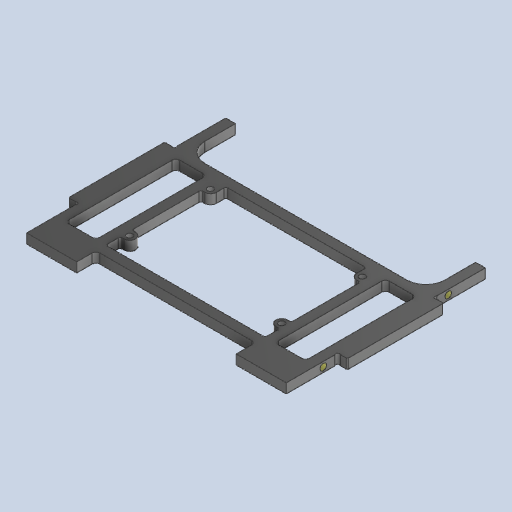
# Autodesk Inventor part: Cockpit_carrier_board_frame
Saved by Autodesk Inventor 2022 (Build 260153000, 153)
## iProperties
Part Number: Cockpit_carrier_board_frame
Material: アセタール樹脂、黒
Document SubType Name: Modeling
Designer: Masato Kubotera
Density: 1.425 g/cm^3
Appearance: 滑らか - 黒
Description: POM T5
Mass: 27.5617 g
Surface Area: 137.943 cm^2
Volume: 19.3415 cm^3
Author: Masato Kubotera
Autodesk Inventor part; units mm, degrees
ref_plane "YZ Plane" through (0, 0, 0) normal (1, 0, 0) x (0, 1, 0)
ref_plane "XZ Plane" through (0, 0, 0) normal (0, 1, 0) x (-1, 0, 0)
derived "Cockpit_side_frame.ipt"
sketch "スケッチ2" plane through (0, 0, 0) normal (0, 1, 0) x (-1, 0, 0)
  line L0 (-23.5, -22.5) -> (-28.5, -27.5)
  line L1 (-28.5, -27.5) -> (-28.5, -91)
  line L2 (-28.5, -91) -> (-23.5, -96)
  line L3 (-23.5, -96) -> (34.25, -96)
  line L4 (36.25, -98) -> (36.25, -131)
  line L5 (36.25, -131) -> (41.25, -136)
  line L6 (41.25, -136) -> (86.5, -136)
  line L7 (91.5, -131) -> (91.5, -20)
  line L8 (91.5, -20) -> (89, -17.5)
  line L9 (89, -17.5) -> (83.25, -17.5)
  line L10 (83.25, -17.5) -> (83.25, -21.0151)
  line L11 (81.7651, -22.5) -> (76.9849, -22.5)
  line L12 (75.5, -21.0151) -> (75.5, -17.5)
  line L13 (75.5, -17.5) -> (67.5, -17.5)
  line L14 (67.5, -17.5) -> (67.5, -21.0151)
  line L15 (66.0151, -22.5) -> (-23.5, -22.5)
  line L16 (-25.25, -25) -> (-20.25, -25) construction
  line L17 (-20.25, -25) -> (-20.25, -93.5) construction
  line L18 (-20.25, -93.5) -> (-25.25, -93.5) construction
  line L19 (-25.25, -93.5) -> (-25.25, -25) construction
  line L20 (-26, -25) -> (-25.25, -25) construction
  line L21 (-25.25, -93.5) -> (-26, -93.5) construction
  line L22 (-26, -93.5) -> (-26, -25) construction
  line L23 (-20.25, -93.5) -> (83.25, -93.5) construction
  line L24 (-20.25, -88.5) -> (83.25, -88.5) construction
  line L25 (83.25, -22.5) -> (83.25, -90.5) construction
  line L26 (83.25, -90.5) -> (88.25, -90.5) construction
  line L27 (88.25, -90.5) -> (88.25, -22.5) construction
  line L28 (83.25, -88.5) -> (83.25, -93.5) construction
  line L29 (83.25, -91) -> (88.25, -91) construction
  line L30 (88.25, -91) -> (88.25, -133.5) construction
  line L31 (83.25, -91) -> (83.25, -133.5) construction
  line L32 (83.25, -133.5) -> (88.25, -133.5) construction
  line L33 (38.75, -133.5) -> (38.75, -128.5) construction
  line L34 (38.75, -128.5) -> (38.75, -93.5) construction
  line L35 (43.75, -93.5) -> (43.75, -128.5) construction
  line L36 (38.75, -128.5) -> (43.75, -128.5) construction
  line L37 (41.25, -128.5) -> (41.25, -93.5) construction
  line L38 (38.75, -128.5) -> (82.1145, -128.5) construction
  line L39 (82.1145, -128.5) -> (82.1145, -133.5) construction
  line L40 (82.1145, -133.5) -> (38.75, -133.5) construction
  line L41 (38.75, -131) -> (82.1145, -131) construction
  line L42 (85.75, -91) -> (85.75, -133.5) construction
  circle A0 centre (85.75, -131) radius 2
  arc A1 (83.25, -128.5) -> (88.25, -128.5) centre (85.75, -131) ccw construction
  line L43 (83.25, -91) -> (-20.25, -91) construction
  line L44 (41.25, -111) -> (43.75, -111) construction
  line L45 (60.4322, -128.5) -> (60.4322, -131) construction
  line L46 (41.2, -115.5651) -> (41.2, -106.4349)
  line L47 (43.8, -107.05) -> (43.8, -114.95)
  line L48 (43.8, -117.05) -> (41.2, -104.95) construction
  line L49 (41.2, -117.05) -> (43.8, -104.95) construction
  line L50 (56.4822, -128.45) -> (64.3822, -128.45)
  line L51 (64.9973, -131.05) -> (55.8672, -131.05)
  line L52 (54.3822, -128.45) -> (66.4822, -131.05) construction
  line L53 (66.4822, -128.45) -> (54.3822, -131.05) construction
  line L54 (41.25, -105) -> (43.75, -105) construction
  line L55 (41.25, -117) -> (43.75, -117) construction
  arc A2 (42.6849, -104.95) -> (41.2, -106.4349) centre (41.9425, -105.6925) ccw
  arc A3 (43.8, -107.05) -> (43.8, -104.95) centre (43.8, -106) ccw
  arc A4 (41.2, -115.5651) -> (42.6849, -117.05) centre (41.9425, -116.3075) ccw
  arc A5 (43.8, -117.05) -> (43.8, -114.95) centre (43.8, -116) ccw
  line L56 (54.4322, -131) -> (54.4322, -128.5) construction
  line L57 (66.4322, -128.5) -> (66.4322, -131) construction
  arc A6 (54.3822, -129.5651) -> (55.8672, -131.05) centre (55.1247, -130.3075) ccw
  arc A7 (56.4822, -128.45) -> (54.3822, -128.45) centre (55.4322, -128.45) ccw
  arc A8 (64.9973, -131.05) -> (66.4822, -129.5651) centre (65.7398, -130.3075) ccw
  arc A9 (66.4822, -128.45) -> (64.3822, -128.45) centre (65.4322, -128.45) ccw
  line L58 (54.3822, -129.5651) -> (54.3822, -128.45)
  line L59 (66.4822, -128.45) -> (66.4822, -129.5651)
  line L60 (42.6849, -104.95) -> (43.8, -104.95)
  line L61 (43.8, -117.05) -> (42.6849, -117.05)
  circle A10 centre (48.4322, -131) radius 1.6
  line L62 (88.25, -22.5) -> (88.25, -17.5) construction
  line L63 (89, -17.5) -> (89, -90.5) construction
  line L64 (89, -90.5) -> (88.25, -90.5) construction
  line L65 (-13.5, -82.5) -> (-13.5, -61)
  arc A11 (-13.5, -82.5) -> (-11.5, -84.5) centre (-11.5, -82.5) ccw
  line L66 (45.5, -84.5) -> (-11.5, -84.5)
  arc A12 (45.5, -84.5) -> (47.5, -82.5) centre (45.5, -82.5) ccw
  line L67 (47.5, -61) -> (47.5, -82.5)
  arc A13 (47.5, -61) -> (45.5, -59) centre (45.5, -61) ccw
  line L68 (-11.5, -59) -> (45.5, -59)
  arc A14 (-11.5, -59) -> (-13.5, -61) centre (-11.5, -61) ccw
  line L69 (31.5, -88.5) -> (31.5, -91) construction
  line L70 (85.75, -22.5) -> (85.75, -90.5) construction
  circle A15 centre (85.75, -34) radius 1.6
  circle A16 centre (85.75, -34) radius 3
  circle A17 centre (85.75, -79) radius 3
  circle A18 centre (85.75, -79) radius 1.6
  line L71 (88.25, -22.5) -> (83.25, -22.5) construction
  arc A19 (88.25, -91) -> (83.25, -91) centre (85.75, -131) ccw construction
  circle A20 centre (48.4322, -131) radius 3
  circle A21 centre (41.25, -99) radius 1.6
  circle A22 centre (41.25, -99) radius 3
  line L72 (6.5, -88.5) -> (6.5, -91) construction
  line L73 (56.5, -88.5) -> (56.5, -91) construction
  line L74 (55.0651, -91.05) -> (7.9349, -91.05)
  line L75 (6.45, -89.5651) -> (6.45, -88.45)
  line L76 (8.55, -88.45) -> (54.45, -88.45)
  line L77 (56.55, -88.45) -> (56.55, -89.5651)
  line L78 (56.55, -91.05) -> (6.45, -88.45) construction
  line L79 (6.45, -91.05) -> (56.55, -88.45) construction
  arc A23 (8.55, -88.45) -> (6.45, -88.45) centre (7.5, -88.45) ccw
  arc A24 (6.45, -89.5651) -> (7.9349, -91.05) centre (7.1925, -90.3075) ccw
  arc A25 (55.0651, -91.05) -> (56.55, -89.5651) centre (55.8075, -90.3075) ccw
  arc A26 (56.55, -88.45) -> (54.45, -88.45) centre (55.5, -88.45) ccw
  line L80 (-20.25, -41) -> (83.25, -41) construction
  line L81 (83.25, -36) -> (-20.25, -36) construction
  line L82 (-20.25, -36) -> (-20.25, -41) construction
  line L83 (-20.25, -38.5) -> (83.25, -38.5) construction
  line L84 (31.5, -41) -> (31.5, -36) construction
  line L85 (55.0651, -35.95) -> (7.9349, -35.95)
  line L86 (7.9349, -41.05) -> (55.0651, -41.05)
  line L87 (56.55, -35.95) -> (6.45, -41.05) construction
  line L88 (6.45, -35.95) -> (55.5877, -40.952) construction
  arc A27 (7.9349, -35.95) -> (6.45, -37.4349) centre (7.1925, -36.6925) ccw
  arc A28 (6.45, -39.5651) -> (7.9349, -41.05) centre (7.1925, -40.3075) ccw
  arc A29 (56.55, -37.4349) -> (55.0651, -35.95) centre (55.8075, -36.6925) ccw
  arc A30 (55.0651, -41.05) -> (56.55, -39.5651) centre (55.8075, -40.3075) ccw
  line L89 (6.5, -41) -> (6.5, -36) construction
  line L90 (56.5, -36) -> (56.5, -41) construction
  line L91 (6.45, -37.4349) -> (6.45, -39.5651)
  line L92 (56.55, -39.5651) -> (56.55, -37.4349)
  circle A31 centre (-1, -38.5) radius 1.6
  circle A32 centre (-1, -38.5) radius 3
  circle A33 centre (64, -38.5) radius 1.6
  circle A34 centre (64, -38.5) radius 3
  line L93 (-25.25, -49.25) -> (-26, -49.25) construction
  line L94 (-25.25, -69.25) -> (-26, -69.25) construction
  line L95 (-26, -59.25) -> (-25.25, -59.25) construction
  line L96 (-22.75, -25) -> (-22.75, -93.5) construction
  arc A35 (66.0151, -22.5) -> (67.5, -21.0151) centre (66.7575, -21.7575) ccw
  arc A36 (75.5, -21.0151) -> (76.9849, -22.5) centre (76.2425, -21.7575) ccw
  line L97 (59.75, -22.5) -> (59.75, -32.5) construction
  line L98 (59.75, -32.5) -> (83.25, -32.5) construction
  line L99 (83.25, -32.5) -> (83.25, -22.5) construction
  line L100 (71.5, -17.5) -> (71.5, -32.5) construction
  line L101 (63.5, -22.5) -> (63.5, -17.5) construction
  line L102 (79.5, -22.5) -> (79.5, -17.5) construction
  circle A37 centre (-22.75, -31.75) radius 1.6
  circle A38 centre (-22.75, -31.75) radius 3
  circle A39 centre (-22.75, -86.75) radius 1.6
  circle A40 centre (-22.75, -86.75) radius 3
  line L103 (67.5, -22.5) -> (75.5, -22.5)
  line L104 (88.25, -17.5) -> (52.5, -17.5) construction
  line L105 (52.5, -17.5) -> (52.5, -22.5) construction
  circle A41 centre (85.75, -98.5) radius 1.475
  circle A42 centre (85.75, -103.5) radius 1.475
  circle A43 centre (85.75, -108.5) radius 1.475
  line L106 (48.25, -93.5) -> (78.75, -93.5)
  line L107 (80.75, -95.5) -> (80.75, -124)
  line L108 (78.75, -126) -> (48.25, -126)
  line L109 (46.25, -124) -> (46.25, -95.5)
  arc A44 (48.25, -93.5) -> (46.25, -95.5) centre (48.25, -95.5) ccw
  arc A45 (46.25, -124) -> (48.25, -126) centre (48.25, -124) ccw
  arc A46 (78.75, -126) -> (80.75, -124) centre (78.75, -124) ccw
  arc A47 (80.75, -95.5) -> (78.75, -93.5) centre (78.75, -95.5) ccw
  arc A48 (36.25, -98) -> (34.25, -96) centre (34.25, -98) ccw
  circle A49 centre (-13.5, -55) radius 1.75
  circle A50 centre (-13.5, -55) radius 2
  line L110 (77.85, -78.65) -> (68.65, -78.65) construction
  line L111 (68.65, -78.65) -> (68.65, -64.85) construction
  line L112 (68.65, -64.85) -> (77.85, -64.85) construction
  line L113 (77.85, -64.85) -> (77.85, -78.65) construction
  line L114 (77.85, -78.65) -> (68.65, -64.85) construction
  line L115 (68.65, -78.65) -> (77.85, -64.85) construction
  line L116 (67.95, -64.2) -> (78.55, -64.2) construction
  line L117 (78.55, -64.2) -> (78.55, -79.3) construction
  line L118 (78.55, -79.3) -> (67.95, -79.3) construction
  line L119 (67.95, -79.3) -> (67.95, -64.2) construction
  line L120 (67.95, -64.2) -> (78.55, -79.3) construction
  line L121 (78.55, -64.2) -> (67.95, -79.3) construction
  line L122 (69.3849, -64.15) -> (77.1151, -64.15)
  line L123 (78.6, -65.6349) -> (78.6, -77.8651)
  line L124 (78.6, -79.35) -> (67.9, -64.15) construction
  line L125 (67.9, -79.35) -> (78.6, -64.15) construction
  line L126 (77.9, -78.7) -> (68.6, -64.8) construction
  line L127 (68.6, -78.7) -> (77.9, -64.8) construction
  arc A51 (69.3849, -64.15) -> (67.9, -65.6349) centre (68.6425, -64.8925) ccw
  arc A52 (70.0849, -64.8) -> (68.6, -66.2849) centre (69.3425, -65.5425) ccw
  line L128 (67.9, -71.75) -> (78.6, -71.75) construction
  line L129 (73.25, -64.15) -> (73.25, -78.7063) construction
  arc A53 (78.6, -65.6349) -> (77.1151, -64.15) centre (77.8575, -64.8925) ccw
  arc A54 (77.9, -66.2849) -> (76.4151, -64.8) centre (77.1575, -65.5425) ccw
  arc A55 (68.6, -77.2151) -> (70.0849, -78.7) centre (69.3425, -77.9575) ccw
  arc A56 (67.9, -77.8651) -> (69.3849, -79.35) centre (68.6425, -78.6075) ccw
  arc A57 (76.4151, -78.7) -> (77.9, -77.2151) centre (77.1575, -77.9575) ccw
  arc A58 (77.1151, -79.35) -> (78.6, -77.8651) centre (77.8575, -78.6075) ccw
  line L130 (70.0849, -64.8) -> (76.4151, -64.8)
  line L131 (77.9, -66.2849) -> (77.9, -77.2151)
  line L132 (67.9, -77.8651) -> (67.9, -65.6349)
  line L133 (68.6, -77.2151) -> (68.6, -66.2849)
  line L134 (76.4151, -78.7) -> (70.0849, -78.7)
  line L135 (77.1151, -79.35) -> (69.3849, -79.35)
  line L136 (-13.5, -71.75) -> (47.5, -71.75) construction
  line L137 (85.75, -56.5) -> (88.25, -56.5) construction
  line L138 (89, -54) -> (88.25, -54) construction
  line L139 (85.7, -69.45) -> (85.7, -43.55)
  line L140 (88.2835, -71.3588) -> (85.7, -41.45) construction
  line L141 (85.7, -71.55) -> (88.3, -41.45) construction
  arc A59 (85.7, -41.45) -> (85.7, -43.55) centre (85.7, -42.5) ccw
  arc A60 (88.3, -42.9349) -> (86.8151, -41.45) centre (87.5575, -42.1925) ccw
  arc A61 (85.7, -69.45) -> (85.7, -71.55) centre (85.7, -70.5) ccw
  arc A62 (86.8151, -71.55) -> (88.3, -70.0651) centre (87.5575, -70.8075) ccw
  line L142 (85.75, -41.5) -> (88.25, -41.5) construction
  line L143 (85.75, -71.5) -> (88.25, -71.5) construction
  arc A63 (89.25, -47.1801) -> (88.3, -46.1348) centre (88.2, -47.1801) ccw
  line L144 (89.25, -47.1801) -> (89.25, -65.8199)
  line L145 (88.25, -46.5) -> (89, -46.5) construction
  line L146 (88.25, -66.5) -> (89, -66.5) construction
  arc A64 (88.3, -66.8652) -> (89.25, -65.8199) centre (88.2, -65.8199) ccw
  line L147 (88.3, -42.9349) -> (88.3, -46.1348)
  line L148 (88.3, -66.8652) -> (88.3, -70.0651)
  line L149 (86.8151, -71.55) -> (85.7, -71.55)
  line L150 (85.7, -41.45) -> (86.8151, -41.45)
  line L151 (86.5, -136) -> (91.5, -131)
  arc A65 (81.7651, -22.5) -> (83.25, -21.0151) centre (82.5075, -21.7575) ccw
  circle A66 centre (85.75, -93.5) radius 2
  circle A67 centre (85.75, -93.5) radius 4 construction
  arc A68 (-24.15, -49.25) -> (-26.25, -49.25) centre (-25.2, -49.25) ccw
  line L152 (-26, -49.25) -> (-26.25, -49.25) construction
  line L153 (-26.25, -49.25) -> (-26.25, -69.25)
  line L154 (-24.15, -49.25) -> (-24.15, -69.25)
  arc A69 (-26.25, -69.25) -> (-24.15, -69.25) centre (-25.2, -69.25) ccw
  point P0 (0, 0)
  point P1 (-25.7227, -96)
  point P2 (-23.5, -22.5)
  point P3 (42.5, -111)
  point P4 (60.4322, -129.75)
  point P5 (31.5, -89.75)
  point P6 (31.5, -38.5)
  point P7 (6.45, -41.05)
  point P8 (52.5, -22)
  point P9 (73.25, -71.75)
  point P10 (73.25, -71.75)
  point P11 (87, -56.5)
  dimension "d1" = 36
  dimension "d2" = 5
  measures "d1" distance from line of L81 point (0, 0)
  measures "d2" distance of L81.end L80.start
ref_plane "作業平面1" through (0, 0, -36) normal (0, 0, 1) x (1, 0, 0)
sketch "スケッチ3" plane through (0, 0, -36) normal (0, 0, 1) x (1, 0, 0)
  line L0 (20.25, -135) -> (20.25, 0)
  line L1 (-83.25, 0) -> (-83.25, -135)
  line L2 (-6.5, 5) -> (-56.5, 5)
  arc A0 (-57.9849, 0) -> (-56.5, 1.4849) centre (-57.2425, 0.7425) ccw
  line L3 (-57.9849, 0) -> (-83.25, 0)
  line L4 (-56.5, 5) -> (-56.5, 1.4849)
  line L5 (-31.5, 0) -> (-31.5, -135) construction
  line L6 (-83.25, -67.5) -> (20.25, -67.5) construction
  arc A1 (-6.5, 1.4849) -> (-5.0151, 0) centre (-5.7575, 0.7425) ccw
  line L7 (20.25, 0) -> (-5.0151, 0)
  line L8 (-6.5, 0) -> (-56.5, 0)
  line L9 (-6.5, 1.4849) -> (-6.5, 5)
  line L10 (-6.5, -140) -> (-56.5, -140)
  arc A2 (-56.5, -136.4849) -> (-57.9849, -135) centre (-57.2425, -135.7425) ccw
  line L11 (-57.9849, -135) -> (-83.25, -135)
  line L12 (-56.5, -140) -> (-56.5, -136.4849)
  arc A3 (-5.0151, -135) -> (-6.5, -136.4849) centre (-5.7575, -135.7425) ccw
  line L13 (20.25, -135) -> (-5.0151, -135)
  line L14 (-6.5, -135) -> (-56.5, -135)
  line L15 (-6.5, -136.4849) -> (-6.5, -140)
  line L16 (-83.25, -130) -> (-67.35, -130)
  line L17 (-57.35, -120) -> (-57.35, -15)
  line L18 (-67.35, -5) -> (-83.25, -5)
  line L19 (3.25, -114) -> (-50.35, -114)
  line L20 (-52.35, -116) -> (-52.35, -128)
  line L21 (-50.35, -130) -> (3.25, -130)
  line L22 (5.25, -128) -> (5.25, -116)
  line L23 (20.25, -109) -> (12.25, -109)
  line L24 (10.25, -107) -> (10.25, -28)
  line L25 (12.25, -26) -> (20.25, -26)
  line L26 (19.25, -24) -> (-51.35, -24) construction
  line L27 (-51.35, -24) -> (-51.35, -111) construction
  line L28 (-51.35, -111) -> (19.25, -111) construction
  line L29 (19.25, -111) -> (19.25, -24) construction
  line L30 (19.25, -24) -> (-51.35, -111) construction
  line L31 (-51.35, -24) -> (19.25, -111) construction
  circle A4 centre (-47.35, -107) radius 1.6
  circle A5 centre (-5.35, -107) radius 1.6
  line L32 (-52.35, -32) -> (-52.35, -103)
  line L33 (-51.35, -104) -> (-47.35, -104)
  line L34 (-44.35, -107) -> (-44.35, -108)
  line L35 (-43.35, -109) -> (-9.35, -109)
  line L36 (-8.35, -108) -> (-8.35, -107)
  line L37 (-2.35, -107) -> (-2.35, -108)
  line L38 (-1.35, -109) -> (4.25, -109)
  line L39 (5.25, -108) -> (5.25, -27)
  arc A6 (-2.35, -107) -> (-8.35, -107) centre (-5.35, -107) ccw
  arc A7 (-44.35, -107) -> (-47.35, -104) centre (-47.35, -107) ccw
  circle A8 centre (-47.35, -28) radius 1.6
  circle A9 centre (-5.35, -28) radius 1.6
  line L40 (-51.35, -31) -> (-47.35, -31)
  line L41 (-44.35, -28) -> (-44.35, -27)
  line L42 (-43.35, -26) -> (-9.35, -26)
  line L43 (-8.35, -27) -> (-8.35, -28)
  line L44 (-2.35, -28) -> (-2.35, -27)
  line L45 (-1.35, -26) -> (4.25, -26)
  arc A10 (-8.35, -28) -> (-2.35, -28) centre (-5.35, -28) ccw
  arc A11 (-47.35, -31) -> (-44.35, -28) centre (-47.35, -28) ccw
  arc A12 (-52.35, -103) -> (-51.35, -104) centre (-51.35, -103) ccw
  arc A13 (-44.35, -108) -> (-43.35, -109) centre (-43.35, -108) ccw
  arc A14 (-9.35, -109) -> (-8.35, -108) centre (-9.35, -108) ccw
  arc A15 (-2.35, -108) -> (-1.35, -109) centre (-1.35, -108) ccw
  arc A16 (4.25, -109) -> (5.25, -108) centre (4.25, -108) ccw
  arc A17 (5.25, -27) -> (4.25, -26) centre (4.25, -27) ccw
  arc A18 (-1.35, -26) -> (-2.35, -27) centre (-1.35, -27) ccw
  arc A19 (-8.35, -27) -> (-9.35, -26) centre (-9.35, -27) ccw
  arc A20 (-43.35, -26) -> (-44.35, -27) centre (-43.35, -27) ccw
  arc A21 (-51.35, -31) -> (-52.35, -32) centre (-51.35, -32) ccw
  arc A22 (-52.35, -128) -> (-50.35, -130) centre (-50.35, -128) ccw
  arc A23 (3.25, -130) -> (5.25, -128) centre (3.25, -128) ccw
  arc A24 (5.25, -116) -> (3.25, -114) centre (3.25, -116) ccw
  arc A25 (-50.35, -114) -> (-52.35, -116) centre (-50.35, -116) ccw
  arc A26 (10.25, -107) -> (12.25, -109) centre (12.25, -107) ccw
  arc A27 (12.25, -26) -> (10.25, -28) centre (12.25, -28) ccw
  line L46 (3.25, -21) -> (-50.35, -21)
  line L47 (-52.35, -19) -> (-52.35, -7)
  line L48 (-50.35, -5) -> (3.25, -5)
  line L49 (5.25, -7) -> (5.25, -19)
  arc A28 (-50.35, -5) -> (-52.35, -7) centre (-50.35, -7) ccw
  arc A29 (5.25, -7) -> (3.25, -5) centre (3.25, -7) ccw
  arc A30 (3.25, -21) -> (5.25, -19) centre (3.25, -19) ccw
  arc A31 (-52.35, -19) -> (-50.35, -21) centre (-50.35, -19) ccw
  arc A32 (-67.35, -130) -> (-57.35, -120) centre (-67.35, -120) ccw
  arc A33 (-57.35, -15) -> (-67.35, -5) centre (-67.35, -15) ccw
  point P0 (0, 0)
  point P1 (-31.5, -67.5)
  point P2 (20.25, 0)
  point P3 (-16.05, -67.5)
  point P4 (-52.35, -104)
  point P5 (-44.35, -109)
  point P6 (-8.35, -109)
  point P7 (-2.35, -109)
  point P8 (5.25, -109)
  point P9 (5.25, -26)
  point P10 (-52.35, -31)
  point P11 (-44.35, -26)
  point P12 (-8.35, -26)
  point P13 (-2.35, -26)
  dimension "d5" = 1.05
  dimension "d6" = 5
  dimension "d7" = 135
  dimension "d17" = 70.6
  dimension "d18" = 87
  dimension "d19" = 3.2
  dimension "d20" = 4
  dimension "d21" = 4
  dimension "d24" = 42
  dimension "d29" = 3
  dimension "d30" = 3
  dimension "d31" = 2
  dimension "d32" = 1
  dimension "d33" = 15
  dimension "d34" = 5
  dimension "d35" = 1
  dimension "d36" = 1
  dimension "d37" = 2
  dimension "d38" = 5
  dimension "d39" = 5
  dimension "d40" = 10
  dimension "d41" = 5
  dimension "d42" = 5
  constraints: 100 end point, 65 point on circle, 40 tangent, 38 symmetric about line, 34 centre point, 30 point on line, 15 equal radius, 14 perpendicular, 8 midpoint, 6 coincident, 6 parallel, 5 horizontal, 4 collinear, 4 vertical, 15 other
  measures "d5" radius of A0
  measures "d6" distance between parallel lines of L8 L2
  measures "d7" distance of L1.start L1.end
  measures "d17" distance of L27.end L28.end
  measures "d18" distance of L26.end L27.end
  measures "d19" diameter of A4
  measures "d20" distance from line of L28 A4.centre
  measures "d21" distance from line of L27 A4.centre
  measures "d24" distance of A4.centre A5.centre
  measures "d29" radius of A7
  measures "d30" radius of A6
  measures "d31" distance between parallel lines of L35 L28
  measures "d32" radius of A12
  measures "d33" distance between parallel lines of L0 L39
  measures "d34" distance between parallel lines of L39 L24
  measures "d35" distance between parallel lines of L0 L29
  measures "d36" distance between parallel lines of L32 L27
  measures "d37" radius of A22
  measures "d38" distance between parallel lines of L35 L19
  measures "d39" distance between parallel lines of L14 L21
  measures "d40" radius of A32
  measures "d41" distance between parallel lines of L11 L16
  measures "d42" distance between parallel lines of L17 L32
extrude "押し出し1" add sketch "スケッチ3" against normal blind 5 contours L13 A3 L14 A2 L11 L1 L16 A32 L17 A33 L18 L3 A0 L8 A1 L7 L0 L25 A27 L24 A26 L23 | A3 L15 L10 L12 A2 L14 | L8 A0 L4 L2 L9 A1
hole "穴1" at (1, 0, -38.5) at (-64, 0, -38.5) direction (0, -1, 0) diameter 3.4587 depth 4 thread size "M4x0.5" class "6H" standard "ANSI Metric M Profile"
ref_plane "作業平面2" through (20.25, -67.5, -36) normal (0, 1, 0) x (1, 0, 0)
mirror "ミラー1" about plane through (20.25, -67.5, -36) normal (0, 1, 0) of "穴1"
chamfer "面取り1" distance 0.5 angle 45 4 edges at (-6.5, -140, -38.5) (-56.5, -140, -38.5) (-6.5, 5, -38.5) (-56.5, 5, -38.5)
equation "\"d21\" = d20"
equation "\"d8\" = d2"
equation "\"d3\" = -d1"
